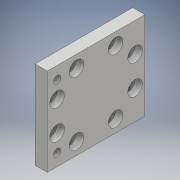
# Autodesk Inventor part: Steam Chest Cover
Saved by Autodesk Inventor 2017 (Build 210142000, 142)
## iProperties
Created: 2018-11-17
Part Number: Steam Chest Cover
Material: Generic
Document SubType Name: Modeling
Designer: Arman Grewal
Density: 1 g/cm^3
Appearance: Default
Author: Arman Grewal
Autodesk Inventor part; units mm, degrees
ref_plane "YZ Plane" through (0, 0, 0) normal (1, 0, 0) x (0, 1, 0)
ref_plane "XZ Plane" through (0, 0, 0) normal (0, 1, 0) x (-1, 0, 0)
ref_plane "XY Plane" through (0, 0, 0) normal (0, 0, 1) x (1, 0, 0)
sketch "Sketch1" plane through (0, 0, 0) normal (1, 0, 0) x (0, 1, 0)
  line L0 (-20, 18) -> (20, 18)
  line L1 (20, 18) -> (20, -18)
  line L2 (20, -18) -> (-20, -18)
  line L3 (-20, -18) -> (-20, 18)
  line L4 (-20, 18) -> (20, -18) construction
  line L5 (20, 18) -> (-20, -18) construction
  circle A0 centre (8, 13) radius 1.75
  circle A1 centre (8, -13) radius 1.75
  line L6 (20, 0) -> (-20, 0) construction
  line L7 (0, 18) -> (0, -18) construction
  circle A2 centre (16, 6) radius 1.75
  circle A3 centre (16, -6) radius 1.75
  circle A4 centre (-8, 13) radius 1.75
  circle A5 centre (-8, -13) radius 1.75
  circle A6 centre (-16, 6) radius 1.75
  circle A7 centre (-16, -6) radius 1.75
  point P0 (0, 0)
  dimension "d0" = 40
  dimension "d1" = 36
  dimension "d2" = 3.5
  dimension "d3" = 3.5
  dimension "d4" = 13
  dimension "d5" = 13
  dimension "d6" = 8
  dimension "d7" = 8
  dimension "d8" = 3.5
  dimension "d9" = 4
  dimension "d10" = 6
  dimension "d11" = 3.5
  dimension "d12" = 6
  dimension "d13" = 4
  constraints: 16 end point, 8 centre point, 6 midpoint, 4 symmetric about line, 2 parallel, 1 horizontal, 1 perpendicular, 4 other
  measures "d0" distance of L1.end L2.end
  measures "d1" distance of L0.end L1.end
  measures "d2" diameter of A0
  measures "d3" diameter of A1
  measures "d4" distance from line of L6 A0.centre
  measures "d5" distance from line of L6 A1.centre
  measures "d6" distance from line of L7 A0.centre
  measures "d7" distance from line of L7 A1.centre
  measures "d8" diameter of A2
  measures "d9" distance from line of L1 A2.centre
  measures "d10" distance from line of L6 A2.centre
  measures "d11" diameter of A3
  measures "d12" distance from line of A3.centre L6
  measures "d13" distance from line of L1 A3.centre
extrude "Extrusion1" add sketch "Sketch1" along normal blind 5
sketch "Sketch2" plane through (5, 0, 0) normal (1, 0, 0) x (0, 0, -1)
  circle A0 centre (-13, 8) radius 1.75 construction
  line L0 (-13, 9.75) -> (-13, 8) construction
  circle A1 centre (-13, 8) radius 3
  circle A2 centre (-6, 16) radius 1.75 construction
  line L1 (-6, 17.75) -> (-6, 16) construction
  circle A3 centre (6, 16) radius 1.75 construction
  line L2 (-6, 16) -> (6, 16) construction
  circle A4 centre (13, 8) radius 1.75 construction
  line L3 (6, 16) -> (13, 8) construction
  circle A5 centre (-6, 16) radius 3
  circle A6 centre (6, 16) radius 3
  circle A7 centre (13, 8) radius 3
  line L4 (-18, 20) -> (-18, -20) construction
  line L5 (-18, 0) -> (18, 0) construction
  line L6 (18, 20) -> (18, -20) construction
  circle A8 centre (-13, -8) radius 3
  circle A9 centre (-6, -16) radius 3
  circle A10 centre (6, -16) radius 3
  circle A11 centre (13, -8) radius 3
  point P0 (0, 0)
  dimension "d16" = 6
  dimension "d17" = 6
  dimension "d18" = 6
  dimension "d19" = 6
  constraints: 10 end point, 8 centre point, 4 coincident, 4 symmetric about line, 2 midpoint, 2 vertical, 2 vertical alignment, 1 perpendicular, 6 other
  measures "d16" diameter of A1
  measures "d17" diameter of A5
  measures "d18" diameter of A6
  measures "d19" diameter of A7
extrude "Extrusion2" cut sketch "Sketch2" against normal blind 3
sketch "Sketch3" plane through (5, 0, 0) normal (1, 0, 0) x (0, 0, -1)
  circle A0 centre (-12.96, -16) radius 1.5
  circle A1 centre (12.96, -16) radius 1.5
  line L0 (0, 0) -> (0, -23.2613) construction
  line L1 (-18, -20) -> (18, -20) construction
  dimension "d22" = 3
  dimension "d23" = 3
  dimension "d24" = 12.96
  dimension "d25" = 12.96
  dimension "d26" = 4
  dimension "d27" = 4
  constraints: 2 centre point, 2 end point, 1 vertical
  measures "d22" diameter of A0
  measures "d23" diameter of A1
  measures "d24" distance from line of L0 A0.centre
  measures "d25" distance from line of L0 A1.centre
  measures "d26" distance from line of L1 A0.centre
  measures "d27" distance from line of L1 A1.centre
extrude "Extrusion3" cut sketch "Sketch3" against normal blind 5
body "Solid1"
